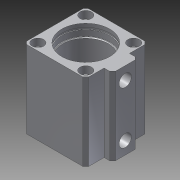
# Autodesk Inventor part: cylinder
Saved by Autodesk Inventor 2016 (Build 200138000, 138)
## iProperties
Created: 2017-06-13
Part Number: cylinder
Material: Aluminum 6061
Document SubType Name: Modeling
Designer: RMcComber
Density: 1 g/cm^3
Appearance: Aluminum - Flat
Author: RMcComber
Autodesk Inventor part; units mm, degrees
ref_plane "YZ Plane" through (0, 0, 0) normal (1, 0, 0) x (0, 1, 0)
sketch "Sketch1" plane through (0, 0, 0) normal (0, 0, 1) x (1, 0, 0)
  line L0 (22, -22) -> (-22, -22)
  line L1 (-22, -22) -> (-22, 22)
  line L2 (-22, 22) -> (22, 22)
  line L3 (22, 22) -> (22, -22)
  line L4 (22, -22) -> (-22, 22) construction
  line L5 (-22, -22) -> (22, 22) construction
  circle A0 centre (0, 0) radius 6
  line L6 (17, -17) -> (-17, -17) construction
  line L7 (-17, -17) -> (-17, 17) construction
  line L8 (-17, 17) -> (17, 17) construction
  line L9 (17, 17) -> (17, -17) construction
  line L10 (17, -17) -> (-17, 17) construction
  line L11 (-17, -17) -> (17, 17) construction
  circle A1 centre (-17, 17) radius 3
  circle A2 centre (17, 17) radius 3
  circle A3 centre (17, -17) radius 3
  circle A4 centre (-17, -17) radius 3
  dimension "d0" = 44
  dimension "d1" = 44
  dimension "d2" = 12
  dimension "d3" = 6
  dimension "d4" = 34
  dimension "d5" = 34
  constraints: 24 end point, 5 centre point, 5 coincident, 4 midpoint, 4 parallel, 3 equal radius, 2 horizontal, 2 perpendicular
  measures "d0" distance of L2.end L0.start
  measures "d1" distance of L0.start L0.end
  measures "d2" diameter of A0
  measures "d3" diameter of A1
  measures "d4" distance of L7.end L8.end
  measures "d5" distance of L8.end L6.start
extrude "Extrusion1" add sketch "Sketch1" along normal blind 55 contours L0 L1 L2 L3 | A0
sketch "Sketch2" plane through (0, 0, 55) normal (0, 0, 1) x (1, 0, 0)
  circle A0 centre (0, 0) radius 16
  dimension "d8" = 32
  constraints: 1 centre point, 1 coincident
  measures "d8" diameter of A0
extrude "Extrusion2" cut sketch "Sketch2" against normal blind 47
sketch "Sketch3" plane through (0, 0, 55) normal (0, 0, 1) x (1, 0, 0)
  circle A0 centre (0, 0) radius 16 projected
  circle A1 centre (0, 0) radius 17
  dimension "d11" = 34
  constraints: 1 centre point, 1 coincident
  measures "d11" diameter of A1
extrude "Extrusion3" cut sketch "Sketch3" against normal blind 8
chamfer "Chamfer1" distance 0.5 angle 45 1 edges at (-16, 0, 47)
ref_plane "Work Plane1" through (0, 0, 51) normal (0, 0, 1) x (1, 0, 0)
sketch "Sketch4" plane through (0, 0, 51) normal (0, 0, 1) x (1, 0, 0)
  circle A0 centre (0, 0) radius 17 projected
  circle A1 centre (-17, -17) radius 3 projected
  circle A2 centre (17, -17) radius 3 projected
  circle A3 centre (17, 17) radius 3 projected
  circle A4 centre (-17, 17) radius 3 projected
  line L0 (-22, -22) -> (22, -22) projected
  line L1 (22, -22) -> (22, 22) projected
  line L2 (22, 22) -> (-22, 22) projected
  line L3 (-22, 22) -> (-22, -22) projected
  circle A5 centre (0, 0) radius 17.5
  dimension "d18" = 35
  constraints: 1 centre point, 1 coincident
  measures "d18" diameter of A5
extrude "Extrusion4" cut sketch "Sketch4" along normal blind 1.5 contours A5
sketch "Sketch5" plane through (0, 0, 55) normal (0, 0, 1) x (1, 0, 0)
  line L0 (22, -22) -> (22, 22) projected
  line L1 (-22, 22) -> (-22, -22) projected
  line L2 (22, 9) -> (28, 9)
  line L3 (28, 9) -> (28, -9)
  line L4 (28, -9) -> (22, -9)
  line L5 (22, -9) -> (22, 9)
  point P0 (22, 0)
  dimension "d21" = 18
  dimension "d22" = 50
  constraints: 8 end point, 2 midpoint, 2 parallel, 1 horizontal, 1 perpendicular
  measures "d21" distance of L2.end L3.end
  measures "d22" distance between parallel lines of L1 L3
extrude "Extrusion5" add sketch "Sketch5" against normal up to surface (55 mm away)
sketch "Sketch6" plane through (28, -9, 55) normal (1, 0, 0) x (0, 0, -1)
  line L0 (0, 0) -> (0, 18) projected
  line L1 (0, 0) -> (55, 0) projected
  line L2 (0, 9) -> (9, 9) construction
  circle A0 centre (9, 9) radius 4.375
  point P0 (55, 9)
  dimension "d25" = 8.75
  dimension "d26" = 9
  constraints: 2 end point, 1 centre point, 1 coincident, 1 midpoint, 1 parallel
  measures "d25" diameter of A0
  measures "d26" distance of L2.start L2.end
extrude "Extrusion6" cut sketch "Sketch6" against normal blind 9
sketch "Sketch7" plane through (28, -9, 55) normal (1, 0, 0) x (0, 0, -1)
  circle A0 centre (9, 9) radius 4.375 projected
  line L0 (0, 0) -> (0, 18) projected
  line L1 (0, 0) -> (55, 0) projected
  line L2 (9, 9) -> (46, 9) construction
  circle A1 centre (46, 9) radius 4.375
  point P0 (55, 9)
  dimension "d29" = 46
  constraints: 2 end point, 1 centre point, 1 coincident, 1 equal radius, 1 parallel
  measures "d29" distance from line of L2.end L0
extrude "Extrusion7" cut sketch "Sketch7" against normal blind 9 contours A1
sketch "Sketch8" plane through (28, -9, 55) normal (1, 0, 0) x (0, 0, -1)
  circle A0 centre (46, 9) radius 4.375 projected
  circle A1 centre (9, 9) radius 4.375 projected
  circle A2 centre (9, 9) radius 1.5
  circle A3 centre (46, 9) radius 1.5
  point P0 (55, 9)
  dimension "d32" = 3
  constraints: 2 centre point, 2 coincident, 1 equal radius
  measures "d32" diameter of A2
extrude "Extrusion8" cut sketch "Sketch8" against normal up to surface contours A2 | A3 round surface about axis through (0, 0, 55) along (0, 0, -1) radius 16 far side no
chamfer "Chamfer2" distance 2 angle 45 6 edges at (22, -22, 27.5) (-22, -22, 27.5) (-22, 22, 27.5) (22, 22, 27.5) (28, -9, 27.5) (28, 9, 27.5)
sketch "Sketch9" plane through (0, 0, 55) normal (0, 0, 1) x (1, 0, 0)
  circle A0 centre (-17, -17) radius 3 projected
  circle A1 centre (17, -17) radius 3 projected
  circle A2 centre (17, 17) radius 3 projected
  circle A3 centre (-17, 17) radius 3 projected
  circle A4 centre (-17, 17) radius 4.1
  circle A5 centre (17, 17) radius 4.1
  circle A6 centre (17, -17) radius 4.1
  circle A7 centre (-17, -17) radius 4.1
  dimension "d38" = 8.2
  constraints: 4 centre point, 4 coincident, 3 equal radius
  measures "d38" diameter of A7
extrude "Extrusion9" cut sketch "Sketch9" against normal blind 5.2 contours A0 | A4 | A5 | A6 | A7
ref_plane "Work Plane2" through (0, 0, 27.5) normal (0, 0, 1) x (1, 0, 0)
mirror "Mirror1" about plane through (0, 0, 27.5) normal (0, 0, 1) of "Extrusion9"
sketch "Sketch10" plane through (17, 17, 49.8) normal (0, 0, 1) x (1, 0, 0)
  point P0 (0, 0)
hole "Hole1" at (17, 17, 49.8) direction (0, 0, -1) diameter 4.917 depth 15.8 tip angle 120 thread size "M6x1" class "6H" standard "ISO Metric profile"
body "Solid1"
